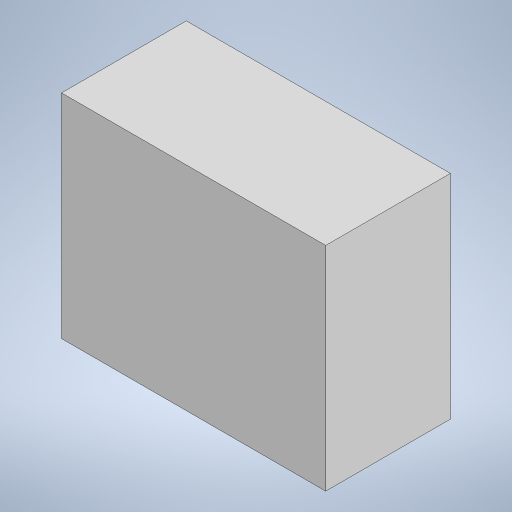
# Autodesk Inventor part: Reflexní optický snímač
Saved by Autodesk Inventor 2023 (Build 270158000, 158)
## iProperties
Created: 2023-01-20
Part Number: Reflexní optický snímač
Material: Všeobecné
Document SubType Name: Modeling
Designer: Kuba
Mass: 0.017748 g
Surface Area: 0.4298 cm^2
Volume: 0.017748 cm^3
Density: 1 g/cm^3
Appearance: Výchozí
Author: Kuba
Autodesk Inventor part; units mm, degrees
ref_plane "YZ Plane" through (0, 0, 0) normal (1, 0, 0) x (0, 1, 0)
ref_plane "XZ Plane" through (0, 0, 0) normal (0, 1, 0) x (-1, 0, 0)
ref_plane "XY Plane" through (0, 0, 0) normal (0, 0, 1) x (1, 0, 0)
sketch "Náčrt1" plane through (0, 0, 0) normal (0, 0, 1) x (1, 0, 0)
  line L0 (0, 0) -> (-1.8, 0) construction
  line L1 (-1.8, 0) -> (-1.8, -1.45) construction
  line L2 (-1.8, -1.45) -> (0, -1.45) construction
  line L3 (0, -1.45) -> (0, 0) construction
  line L4 (-1.8, -1.45) -> (1.8, -1.45)
  line L5 (1.8, -1.45) -> (1.8, 1.45)
  line L6 (1.8, 1.45) -> (-1.8, 1.45)
  line L7 (-1.8, 1.45) -> (-1.8, -1.45)
  dimension "d0" = 1.8
  dimension "d1" = 1.45
  dimension "d2" = 3.6
  dimension "d3" = 2.9
  constraints: 16 end point, 4 parallel, 2 horizontal, 2 perpendicular
  measures "d0" distance of L2.end L1.end
  measures "d1" distance of L1.end L0.end
  measures "d2" distance of L6.end L5.end
  measures "d3" distance of L5.end L4.end
extrude "Vysunutí1" add sketch "Náčrt1" along normal blind 1.7
